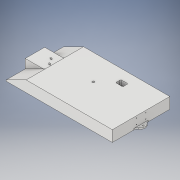
# Autodesk Inventor part: Enclosure_v2
Saved by Autodesk Inventor 2019 (Build 230136000, 136)
## iProperties
Created: 2020-02-14
Part Number: Enclosure_v2
Material: Generic
Document SubType Name: Modeling
Designer: close
Density: 1 g/cm^3
Appearance: Smooth - White
Author: close
Autodesk Inventor part; units mm, degrees
ref_plane "YZ Plane" through (0, 0, 0) normal (1, 0, 0) x (0, 1, 0)
ref_plane "XZ Plane" through (0, 0, 0) normal (0, 1, 0) x (-1, 0, 0)
ref_plane "XY Plane" through (0, 0, 0) normal (0, 0, 1) x (1, 0, 0)
sketch "Sketch1" plane through (0, 0, 0) normal (0, 1, 0) x (-1, 0, 0)
  line L0 (0, 0) -> (240, 0)
  line L1 (240, 0) -> (240, -130)
  line L2 (240, -130) -> (0, -130)
  line L3 (0, -130) -> (0, 0)
  dimension "d0" = 130
  dimension "d1" = 240
  constraints: 8 end point, 2 parallel, 1 horizontal, 1 perpendicular
  measures "d0" distance between parallel lines of L2 L0
  measures "d1" distance between parallel lines of L3 L1
extrude "Main Rectangular Prism" add sketch "Sketch1" along normal blind 25
sketch "Sketch2" plane through (0, 0, 0) normal (0, -1, 0) x (1, 0, 0)
  line L0 (-5, -111) -> (-105, -111) construction
  line L1 (-105, -111) -> (-105, -32) construction
  line L2 (-105, -32) -> (-5, -32) construction
  line L3 (-5, -32) -> (-5, -111) construction
  line L4 (-15, -94) -> (-101, -94) construction
  line L5 (-101, -94) -> (-101, -36) construction
  line L6 (-101, -36) -> (-15, -36) construction
  line L7 (-15, -36) -> (-15, -94) construction
  line L8 (-103.25, -76.2) -> (-99.35, -76.2) construction
  line L9 (-99.35, -76.2) -> (-99.35, -53.8) construction
  line L10 (-99.35, -53.8) -> (-103.25, -53.8) construction
  line L11 (-103.25, -53.8) -> (-103.25, -76.2) construction
  line L12 (0, 0) -> (-240, 0) construction
  line L13 (-240, -130) -> (0, -130) construction
  line L14 (-2.5, -113) -> (-107.5, -113)
  line L15 (-107.5, -113) -> (-107.5, -29)
  line L16 (-107.5, -29) -> (-2.5, -29)
  line L17 (-2.5, -29) -> (-2.5, -113)
  line L18 (0, -130) -> (0, 0) projected
  dimension "d5" = 100
  dimension "d6" = 86
  dimension "d7" = 58
  dimension "d8" = 79
  dimension "d9" = 4
  dimension "d10" = 4
  dimension "d12" = 22.4
  dimension "d13" = 17.8
  dimension "d14" = 130
  dimension "d16" = 53.8
  dimension "d17" = 3.9
  dimension "d18" = 1.75
  dimension "d19" = 105
  dimension "d20" = 2.5
  dimension "d21" = 84
  dimension "d22" = 2
  dimension "d25" = 2.5
  constraints: 32 end point, 8 parallel, 4 horizontal, 4 perpendicular
  measures "d5" distance of L0.start L0.end
  measures "d6" distance of L4.start L4.end
  measures "d7" distance of L6.end L4.start
  measures "d8" distance of L2.end L0.start
  measures "d9" distance between parallel lines of L2 L6
  measures "d10" distance between parallel lines of L1 L5
  measures "d12" distance between parallel lines of L10 L8
  measures "d13" distance from line of L5.end L10
  measures "d14" distance between parallel lines of L12 L13
  measures "d16" distance between parallel lines of L13 L8
  measures "d17" distance between parallel lines of L11 L9
  measures "d18" distance between parallel lines of L1 L11
  measures "d19" distance of L14.start L14.end
  measures "d20" distance between parallel lines of L18 L17
  measures "d21" distance between parallel lines of L16 L14
  measures "d22" distance between parallel lines of L0 L14
  measures "d25" distance between parallel lines of L17 L3
sketch "Sketch21" plane through (0, 0, 0) normal (0, -1, 0) x (1, 0, 0)
  line L0 (5, -65) -> (-228, -65) construction
  line L1 (-228, -81) -> (-228, -49) construction
  line L2 (-240, -130) -> (0, -130) construction
  line L3 (0, 0) -> (-240, 0) construction
  line L4 (-240, 0) -> (-240, -130) construction
  dimension "d221" = 233
  dimension "d222" = 32
  dimension "d223" = 130
  dimension "d224" = 65
  dimension "d225" = 12
  constraints: 4 end point, 1 horizontal, 1 midpoint, 1 vertical
  measures "d221" distance of L0.start L0.end
  measures "d222" distance of L1.end L1.start
  measures "d223" distance between parallel lines of L2 L3
  measures "d224" distance from line of L0.start L2
  measures "d225" distance between parallel lines of L4 L1
sketch "Sketch22" plane through (0, 25, 0) normal (0, 1, 0) x (1, 0, 0)
  line L0 (-240, 0) -> (-240, 130) projected
  line L1 (-195, 0) -> (-195, 130) projected
  line L2 (-240, 87) -> (-195, 87)
  line L3 (-195, 87) -> (-195, 43)
  line L4 (-195, 43) -> (-240, 43)
  line L5 (-240, 43) -> (-240, 87)
  line L6 (-195, 130) -> (-240, 130) projected
  point P0 (0, 0)
  dimension "d226" = 44
  dimension "d227" = 130
  dimension "d228" = 43
  constraints: 8 end point, 2 parallel, 2 point on line, 1 horizontal, 1 perpendicular
  measures "d226" distance between parallel lines of L4 L2
  measures "d227" distance of L0.start L0.end
  measures "d228" distance between parallel lines of L2 L6
extrude "2mm indent" cut sketch "Sketch22" against normal blind 2 contours L0 L2 L1 L4
sketch "Sketch23" plane through (0, 0, 0) normal (0, -1, 0) x (1, 0, 0)
  line L0 (0, 0) -> (0, -130) projected
  arc A0 (0, -76.619) -> (0, -53.381) centre (-3, -65) ccw
  line L1 (-240, -130) -> (0, -130) projected
  point P0 (0, -115)
  dimension "d231" = 65
  dimension "d232" = 3
  dimension "d233" = 12
  constraints: 2 point on circle, 2 point on line, 1 centre point
  measures "d231" distance from line of L1 A0.centre
  measures "d232" distance from line of L0 A0.centre
  measures "d233" radius of A0
extrude "Extrusion26" add sketch "Sketch23" against normal blind 3
fillet "Rear mount fillet" radius 7 2 edges at (0, 1.5, -76.619) (0, 1.5, -53.381)
sketch "Sketch45" plane through (-240, 0, 0) normal (0, 0, 1) x (1, 0, 0)
  line L0 (45, 25) -> (0, 2.5)
  line L1 (0, 0) -> (0, 25) projected
  line L2 (0, 25) -> (0, 2.5)
  line L3 (0, 25) -> (240, 25) projected
  line L4 (45, 25) -> (0, 25)
  point P0 (240, 0)
  dimension "d590" = 2.5
  constraints: 6 end point, 2 collinear, 1 point on line
  measures "d590" distance of L1.start L0.end
extrude "Slope Left" cut sketch "Sketch45" against normal up to surface (43 mm away)
sketch "Sketch46" plane through (0, 0, -130) normal (0, 0, -1) x (-1, 0, 0)
  line L0 (195, 25) -> (240, 25) projected
  line L1 (240, 0) -> (240, 25) projected
  line L2 (195, 25) -> (240, 2.5) projected
  point P0 (0, 0)
extrude "Slope Right" cut sketch "Sketch46" against normal up to surface (43 mm away)
hole "Hole5" at (5, 0, -65) at (-228, 0, -81) at (-228, 0, -49) direction (0, 1, 0) diameter 3.4 depth 8.8 clearance for "Flat Head Machine Screw" size "M3" standard "Ansi Metric M Profile"
sketch "Sketch24" plane through (0, 23, 0) normal (0, 1, 0) x (1, 0, 0)
  line L0 (-201.625, 59) -> (-199.375, 59) construction
  line L1 (-201.625, 60.125) -> (-199.375, 60.125)
  line L2 (-199.375, 57.875) -> (-201.625, 57.875)
  arc A0 (-201.625, 60.125) -> (-201.625, 57.875) centre (-201.625, 59) ccw
  arc A1 (-199.375, 57.875) -> (-199.375, 60.125) centre (-199.375, 59) ccw
  line L3 (-208.375, 71) -> (-210.625, 71) construction
  line L4 (-208.375, 72.125) -> (-210.625, 72.125)
  line L5 (-210.625, 69.875) -> (-208.375, 69.875)
  arc A2 (-208.375, 69.875) -> (-208.375, 72.125) centre (-208.375, 71) ccw
  arc A3 (-210.625, 72.125) -> (-210.625, 69.875) centre (-210.625, 71) ccw
  line L6 (-195, 87) -> (-195, 43) projected
  circle A4 centre (5, 65) radius 1.7 projected
  point P0 (0, 0)
  point P1 (-205, 65)
  point P2 (-200.5, 59)
  point P3 (-209.5, 71)
  dimension "d244" = 2.25
  dimension "d245" = 2.25
  dimension "d246" = 2.25
  dimension "d247" = 2.25
  dimension "d248" = 12
  dimension "d249" = 6
  dimension "d250" = 9
  dimension "d251" = 4.5
  dimension "d255" = 10
  dimension "d589" = 210
  constraints: 16 end point, 8 point on circle, 8 tangent, 4 centre point, 3 parallel, 2 midpoint, 1 horizontal
  measures "d244" distance of L3.start L3.end
  measures "d245" distance of L0.start L0.end
  measures "d246" distance between parallel lines of L2 L1
  measures "d247" distance between parallel lines of L5 L4
  measures "d248" distance between parallel lines of L0 L3
  measures "d249" distance from line of point (-205, 65) L0
  measures "d250" horizontal distance of point (-209.5, 71) point (-200.5, 59)
  measures "d251" horizontal distance of point (-200.5, 59) point (-205, 65)
  measures "d255" distance from line of L6 point (-205, 65)
  measures "d589" distance of A4.centre point (-205, 65)
extrude "Extrusion27" add sketch "Sketch24" along normal blind 2 contours L1 A1 L2 A0 | A2 L5 A3 L4
shell "Shell1" [suppressed]
sketch "Sketch27" plane through (-192.7649, 23, -128) normal (0, -1, 0) x (1, 0, 0)
  line L0 (186.2649, 18.5) -> (100.2649, 18.5) construction
  line L1 (100.2649, 18.5) -> (100.2649, 76.5) construction
  line L2 (100.2649, 76.5) -> (186.2649, 76.5) construction
  line L3 (186.2649, 76.5) -> (186.2649, 18.5) construction
  line L4 (190.2649, 1.5) -> (90.2649, 1.5) construction
  line L5 (90.2649, 1.5) -> (90.2649, 80.5) construction
  line L6 (90.2649, 80.5) -> (190.2649, 80.5) construction
  line L7 (190.2649, 80.5) -> (190.2649, 1.5) construction
  line L8 (60.9002, 126.8579) -> (96.9002, 126.8579) construction
  line L9 (38.0929, 36.45) -> (10.1929, 36.45) construction
  line L10 (190.7649, 0) -> (-45.2351, 0) construction
  line L11 (190.7649, 46.8445) -> (190.7649, 0) construction
  circle A0 centre (186.2649, 18.5) radius 3
  circle A1 centre (100.2649, 18.5) radius 3
  circle A2 centre (186.2649, 76.5) radius 3
  circle A3 centre (100.2649, 76.5) radius 3
  line L12 (186.2649, 15.5) -> (190.7649, 15.5)
  line L13 (186.2649, 21.5) -> (190.7649, 21.5)
  line L14 (190.7649, 15.5) -> (190.7649, 21.5)
  line L15 (186.2649, 73.5) -> (190.7649, 73.5)
  line L16 (190.7649, 126) -> (190.7649, 0) projected
  line L17 (186.2649, 79.5) -> (190.7649, 79.5)
  line L18 (190.7649, 73.5) -> (190.7649, 79.5)
  line L19 (192.7649, 79.1555) -> (192.7649, 128) projected
  point P0 (53.2929, 87.25)
  point P1 (5.0929, 88.55)
  point P2 (38.0929, 36.45)
  point P3 (-1.349, 0)
  point P4 (0.8663, 0)
  dimension "d288" = 100
  dimension "d289" = 79
  dimension "d290" = 86
  dimension "d291" = 58
  dimension "d298" = 1.3
  dimension "d299" = 27.9
  dimension "d300" = 5.1
  dimension "d301" = 50.8
  dimension "d303" = 4
  dimension "d304" = 4
  dimension "d305" = 1.5
  dimension "d306" = 0.5
  dimension "d307" = 6
  dimension "d309" = 6
  dimension "d310" = 6
  dimension "d556" = 187.672
  dimension "d557" = 6
  dimension "d564" = 15.2
  dimension "d565" = 88.55
  constraints: 32 end point, 10 coincident, 6 perpendicular, 6 point on line, 5 parallel, 4 centre point, 4 point on circle, 3 horizontal, 3 tangent, 1 collinear
  measures "d288" distance of L4.start L4.end
  measures "d289" distance of L6.end L4.start
  measures "d290" distance of L0.start L0.end
  measures "d291" distance of L2.end L0.start
  measures "d298" vertical distance of point (5.093, 88.55) point (53.293, 87.25)
  measures "d299" distance of L9.start L9.end
  measures "d300" horizontal distance of point (5.093, 88.55) point (10.193, 36.45)
  measures "d301" vertical distance of point (38.093, 36.45) point (53.293, 87.25)
  measures "d303" distance between parallel lines of L7 L3
  measures "d304" distance between parallel lines of L6 L2
  measures "d305" distance between parallel lines of L10 L4
  measures "d306" distance between parallel lines of L11 L7
  measures "d307" diameter of A0
  measures "d309" diameter of A2
  measures "d310" diameter of A3
  measures "d556" distance from line of L19 point (5.093, 88.55)
  measures "d557" diameter of A1
  measures "d564" horizontal distance of point (38.093, 36.45) point (53.293, 87.25)
  measures "d565" distance from line of L10 point (5.093, 88.55)
extrude "Extrusion30" [suppressed]
sketch "Sketch28" plane through (-192.7649, 3, -128) normal (0, -1, 0) x (1, 0, 0)
  arc A0 (186.2649, 21.5) -> (186.2649, 15.5) centre (186.2649, 18.5) ccw construction
  arc A1 (186.2649, 79.5) -> (186.2649, 73.5) centre (186.2649, 76.5) ccw construction
  circle A2 centre (100.2649, 76.5) radius 3 construction
  circle A3 centre (100.2649, 18.5) radius 3 construction
  arc A4 (186.2649, 79.5) -> (186.2649, 73.5) centre (186.2649, 76.5) ccw construction
  circle A5 centre (100.2649, 18.5) radius 3 construction
  point P0 (192.7649, 128)
  point P1 (186.2649, 18.5)
  point P2 (100.2649, 18.5)
  constraints: 4 coincident
hole "Hole7" [suppressed]
sketch "Sketch29" plane through (0, 25, 0) normal (0, 1, 0) x (1, 0, 0)
  line L0 (-81, 47.55) -> (-20, 47.55)
  line L1 (-20, 47.55) -> (-20, 88.55)
  line L2 (-81, 88.55) -> (-81, 47.55)
  line L3 (-79.85, 48.5) -> (-21.15, 48.5) construction
  line L4 (-21.15, 87.6) -> (-79.85, 87.6) construction
  line L5 (-79.85, 87.6) -> (-79.85, 80.3462) construction
  line L6 (-21.15, 87.6) -> (-21.15, 80.3462) construction
  line L7 (-5.3, 69.5) -> (-8.15, 69.5)
  line L8 (-8.15, 91.5) -> (-5.3, 91.5)
  line L9 (-8.15, 69.5) -> (-8.15, 91.5)
  line L10 (-5.3, 91.5) -> (-5.3, 69.5)
  line L11 (-66, 91.55) -> (-66, 91.55)
  line L12 (-63.8038, 91.55) -> (-58.1962, 91.55)
  line L13 (-56, 91.55) -> (-56, 91.55)
  line L14 (-20, 88.55) -> (-53, 88.55)
  line L15 (-69, 88.55) -> (-81, 88.55)
  arc A0 (-55.5981, 90.05) -> (-53, 88.55) centre (-53, 91.55) ccw
  arc A1 (-69, 88.55) -> (-66.4019, 90.05) centre (-69, 91.55) ccw
  arc A2 (-63.8038, 91.55) -> (-66.4019, 90.05) centre (-63.8038, 88.55) ccw
  arc A3 (-55.5981, 90.05) -> (-58.1962, 91.55) centre (-58.1962, 88.55) ccw
  point P0 (0, 0)
  dimension "d323" = 41
  dimension "d320" = 39.1
  dimension "d321" = 58.7
  dimension "d322" = 61
  dimension "d324" = 0.95
  dimension "d325" = 1.15
  dimension "d558" = 41
  dimension "d559" = 41
  dimension "d560" = 3
  dimension "d561" = 10
  dimension "d562" = 15
  dimension "d563" = 3
  constraints: 32 end point, 10 point on circle, 8 tangent, 5 horizontal, 5 parallel, 4 centre point, 3 equal radius, 3 vertical, 2 point on line, 1 perpendicular, 10 other
  measures "d320" distance between parallel lines of L4 L3
  measures "d321" distance of L4.start L4.end
  measures "d322" distance of L1.end L2.start
  measures "d324" distance between parallel lines of L3 L0
  measures "d325" distance between parallel lines of L5 L2
  measures "d558" distance between parallel lines of L0 L14
  measures "d559" distance between parallel lines of L0 L15
  measures "d560" distance between parallel lines of L15 L12
  measures "d561" distance of L11.end L13.start
  measures "d562" distance between parallel lines of L2 L11
  measures "d563" radius of A0
extrude "Extrusion31" [suppressed]
fillet "Fillet5" [suppressed]
sketch "Sketch30" plane through (0, 0, -130) normal (1, 0, 0) x (0, 0, -1)
  line L0 (-77.5, 31) -> (-52.5, 31) construction
  line L1 (-52.5, 31) -> (-52.5, 6) construction
  line L2 (-52.5, 6) -> (-77.5, 6) construction
  line L3 (-77.5, 6) -> (-77.5, 31) construction
  line L4 (-75.5, 20.5) -> (-54.5, 20.5) construction
  line L5 (-54.5, 20.5) -> (-54.5, 8) construction
  line L6 (-54.5, 8) -> (-75.5, 8) construction
  line L7 (-75.5, 8) -> (-75.5, 20.5) construction
  line L8 (-130, 25) -> (0, 25) construction
  line L9 (0, 0) -> (0, 25) construction
  line L10 (-130, 0) -> (-130, 25) construction
  line L11 (-72, 23) -> (-58, 23)
  line L12 (-56, 21) -> (-56, 11)
  line L13 (-58, 9) -> (-72, 9)
  line L14 (-74, 11) -> (-74, 21)
  arc A0 (-72, 23) -> (-74, 21) centre (-72, 21) ccw
  arc A1 (-74, 11) -> (-72, 9) centre (-72, 11) ccw
  arc A2 (-58, 9) -> (-56, 11) centre (-58, 11) ccw
  arc A3 (-56, 21) -> (-58, 23) centre (-58, 21) ccw
  point P0 (-74, 23)
  point P1 (-56, 9)
  point P2 (-56, 23)
  point P3 (-74, 9)
  dimension "d329" = 25
  dimension "d330" = 25
  dimension "d331" = 6
  dimension "d332" = 12.5
  dimension "d333" = 21
  dimension "d334" = 2
  dimension "d335" = 2
  dimension "d336" = 130
  dimension "d337" = 52.5
  dimension "d338" = 18
  dimension "d339" = 14
  dimension "d340" = 3.5
  dimension "d341" = 8
  dimension "d351" = 2
  constraints: 24 end point, 8 point on circle, 8 point on line, 8 tangent, 6 parallel, 4 centre point, 4 coincident, 3 equal radius, 3 horizontal, 3 perpendicular
  measures "d329" distance of L0.end L1.end
  measures "d330" distance of L0.start L0.end
  measures "d331" distance between parallel lines of L8 L0
  measures "d332" distance of L4.end L5.end
  measures "d333" distance of L5.end L6.end
  measures "d334" distance between parallel lines of L1 L5
  measures "d335" distance between parallel lines of L2 L6
  measures "d336" distance between parallel lines of L9 L10
  measures "d337" distance between parallel lines of L3 L10
  measures "d338" distance of point (-74, 23) point (-56, 23)
  measures "d339" distance between parallel lines of L13 L11
  measures "d340" distance between parallel lines of L3 L14
  measures "d341" distance between parallel lines of L0 L11
  measures "d351" radius of A0
extrude "Extrusion32" [suppressed]
hole "Hole8" at (0, 20.5, -54.5) at (0, 8, -54.5) at (0, 8, -75.5) at (0, 20.5, -75.5) direction (-1, 0, 0) diameter 1.567 depth 6.3 thread size "M2x0.4" class "6H" standard "ANSI Metric M Profile"
sketch "Sketch31" plane through (-194.1139, 0, -128) normal (0, 0, 1) x (1, 0, 0)
  line L0 (-43.8861, 23) -> (192.1139, 23) construction
  line L1 (192.1139, 0) -> (192.1139, 23) construction
  line L2 (-43.8861, 0) -> (192.1139, 0) construction
  circle A0 centre (185.5918, 9.5024) radius 3
  arc A1 (122.6139, 16.45) -> (122.4139, 16.65) centre (122.4139, 16.45) ccw construction
  line L3 (106.7139, 16.4) -> (106.7139, 3.35)
  line L4 (122.6139, 16.45) -> (122.6139, 16.6499)
  line L5 (122.6139, 16.6499) -> (122.4139, 16.65)
  line L6 (122.6139, 16.6499) -> (106.7139, 16.6499)
  line L7 (106.7139, 16.6499) -> (106.7139, 3.35)
  line L8 (106.7139, 3.35) -> (122.6139, 3.35)
  line L9 (122.6139, 3.35) -> (122.6139, 16.6499)
  arc A2 (126.0639, 18.47) -> (125.4639, 17.87) centre (126.0639, 17.87) ccw construction
  arc A3 (125.4639, 4.85) -> (126.0639, 4.25) centre (126.0639, 4.85) ccw construction
  arc A4 (138.5639, 17.87) -> (137.9639, 18.47) centre (137.9639, 17.87) ccw construction
  line L10 (138.5639, 17.87) -> (138.5639, 18.47) construction
  line L11 (138.5639, 18.47) -> (137.9639, 18.47) construction
  line L12 (126.0639, 18.47) -> (125.4639, 18.47) construction
  line L13 (125.4639, 18.47) -> (125.4639, 17.87) construction
  line L14 (125.4639, 4.85) -> (125.4639, 4.25) construction
  line L15 (125.4639, 4.25) -> (126.0639, 4.25) construction
  line L16 (138.5639, 18.47) -> (125.4639, 18.47)
  line L17 (125.4639, 18.47) -> (125.4639, 12.75)
  line L18 (125.4639, 12.75) -> (138.5639, 12.75)
  line L19 (138.5639, 12.75) -> (138.5639, 18.47)
  line L20 (155.5639, 12.75) -> (155.5639, 18.47)
  line L21 (155.5639, 18.47) -> (142.4639, 18.47)
  line L22 (142.4639, 18.47) -> (142.4639, 12.75)
  line L23 (142.4639, 12.75) -> (155.5639, 12.75)
  line L24 (138.5639, 4.25) -> (138.5639, 9.97)
  line L25 (138.5639, 9.97) -> (125.4639, 9.97)
  line L26 (125.4639, 9.97) -> (125.4639, 4.25)
  line L27 (125.4639, 4.25) -> (138.5639, 4.25)
  line L28 (155.5639, 4.25) -> (155.5639, 9.97)
  line L29 (155.5639, 9.97) -> (142.4639, 9.97)
  line L30 (142.4639, 9.97) -> (142.4639, 4.25)
  line L31 (142.4639, 4.25) -> (155.5639, 4.25)
  arc A5 (176.3139, 20.3762) -> (175.5139, 21.1762) centre (175.5139, 20.3762) ccw
  arc A6 (176.1088, 17.2149) -> (176.31, 17.6362) centre (175.6139, 17.7099) ccw
  arc A7 (160.2139, 21.1762) -> (159.4201, 20.4762) centre (160.2139, 20.3762) ccw
  line L32 (175.5139, 21.1762) -> (160.2139, 21.1762)
  arc A8 (159.4211, 16.2162) -> (160.1139, 15.6162) centre (160.1139, 16.3162) ccw
  arc A9 (174.2102, 15.6062) -> (174.7051, 15.8112) centre (174.2102, 16.3062) ccw
  line L33 (176.31, 17.6362) -> (176.3139, 20.3762)
  line L34 (176.1088, 17.2149) -> (174.7051, 15.8112)
  line L35 (174.2102, 15.6062) -> (160.1139, 15.6162)
  line L36 (159.4211, 16.2162) -> (159.4201, 20.4762)
  line L37 (-43.8861, 23) -> (192.1139, 23) projected
  line L38 (192.1139, 0) -> (192.1139, 23) projected
  line L39 (-43.8861, 0) -> (192.1139, 0) projected
  arc A10 (175.3629, 8.3762) -> (174.5629, 9.1762) centre (174.5629, 8.3762) ccw
  arc A11 (161.1629, 9.1762) -> (160.3629, 8.3762) centre (161.1629, 8.3762) ccw
  arc A12 (160.3629, 5.8978) -> (160.9276, 5.1331) centre (161.1629, 5.8978) ccw
  arc A13 (161.6118, 4.8762) -> (161.4748, 4.9648) centre (161.3866, 4.678) ccw
  arc A14 (162.4729, 3.8977) -> (163.0735, 3.6262) centre (163.0735, 4.4262) ccw
  arc A15 (172.6523, 3.6262) -> (173.2528, 3.8977) centre (172.6523, 4.4262) ccw
  arc A16 (174.2509, 4.9648) -> (174.1139, 4.8762) centre (174.3391, 4.678) ccw
  arc A17 (174.7981, 5.1331) -> (175.3629, 5.8978) centre (174.5629, 5.8978) ccw
  line L40 (174.5629, 9.1762) -> (161.1629, 9.1762)
  line L41 (160.3629, 8.3762) -> (160.3629, 5.8978)
  line L42 (160.9276, 5.1331) -> (161.4748, 4.9648)
  line L43 (161.6118, 4.8762) -> (162.4729, 3.8977)
  line L44 (163.0735, 3.6262) -> (172.6523, 3.6262)
  line L45 (174.1139, 4.8762) -> (173.2528, 3.8977)
  line L46 (174.7981, 5.1331) -> (174.2509, 4.9648)
  line L47 (175.3629, 8.3762) -> (175.3629, 5.8978)
  line L48 (-43.8861, 0) -> (-43.8861, 23) projected
  line L49 (-43.8861, 0) -> (-43.8861, 23) projected
  point P0 (194.1139, 0)
  dimension "d360" = 6
  dimension "d416" = 6.5221
  dimension "d473" = 17
  dimension "d476" = 8.5
  dimension "d479" = 0
  constraints: 84 end point, 34 point on circle, 18 centre point, 9 perpendicular, 9 tangent, 6 horizontal, 4 parallel, 3 vertical, 2 collinear, 1 point on line, 92 other
  measures "d360" diameter of A0
  measures "d416" distance from line of A0.centre L1
  measures "d473" distance of L18.end L20.start
  measures "d476" distance of L18.end L24.start
  measures "d479" distance between parallel lines of L15 L27
extrude "Extrusion33" [suppressed]
sketch "Sketch32" plane through (0, 25, 0) normal (0, 1, 0) x (1, 0, 0)
  line L0 (-74.17, 95.83) -> (-86.33, 95.83)
  line L1 (-88.33, 97.83) -> (-88.33, 105.63)
  line L2 (-86.33, 107.63) -> (-74.17, 107.63)
  line L3 (-72.17, 105.63) -> (-72.17, 97.83)
  arc A0 (-74.17, 95.83) -> (-72.17, 97.83) centre (-74.17, 97.83) ccw
  arc A1 (-72.17, 105.63) -> (-74.17, 107.63) centre (-74.17, 105.63) ccw
  arc A2 (-86.33, 107.63) -> (-88.33, 105.63) centre (-86.33, 105.63) ccw
  arc A3 (-88.33, 97.83) -> (-86.33, 95.83) centre (-86.33, 97.83) ccw
  point P0 (0, 0)
  point P1 (-75.17, 104.63)
  point P2 (-85.33, 104.63)
  point P3 (-85.33, 98.83)
  point P4 (-75.17, 98.83)
  dimension "d480" = 2
  dimension "d481" = 3
  dimension "d482" = 3
  dimension "d483" = 3
  dimension "d484" = 3
  constraints: 8 end point, 8 point on circle, 8 tangent, 4 centre point, 3 equal radius, 2 parallel, 1 horizontal, 1 perpendicular, 4 other
  measures "d480" radius of A0
  measures "d481" distance from line of L3 point (-75.17, 98.83)
  measures "d482" distance from line of point (-85.33, 98.83) L0
  measures "d483" distance from line of point (-85.33, 98.83) L1
  measures "d484" distance from line of L2 point (-85.33, 104.63)
extrude "Extrusion34" cut sketch "Sketch32" against normal blind 10
sketch "Sketch33" plane through (0, 25, 0) normal (0, 1, 0) x (1, 0, 0)
  circle A0 centre (-128.5, 111.25) radius 1.2295 construction
  circle A1 centre (-99.5, 111.25) radius 1.2295 construction
  circle A2 centre (-99.5, 58.75) radius 1.2295 construction
  circle A3 centre (-128.5, 58.75) radius 1.2295 construction
  circle A4 centre (-102.1923, 37.5) radius 2.25 construction
  circle A5 centre (-102.1923, 6) radius 2.25 construction
  circle A6 centre (-7.1923, 37.5) radius 2.25 construction
  circle A7 centre (-7.1923, 6) radius 2.25 construction
  circle A8 centre (-126.2337, 102.7663) radius 1.7399 construction
  circle A9 centre (-126.2337, 67.4838) radius 1.7399 construction
  circle A10 centre (-115.03, 72.27) radius 1.095 construction
  line L0 (-117.7, 74) -> (-131.7, 74)
  line L1 (-131.7, 74) -> (-131.7, 96.5)
  line L2 (-131.7, 96.5) -> (-117.7, 96.5)
  line L3 (-117.7, 96.5) -> (-117.7, 74)
  circle A11 centre (-126.2337, 67.4838) radius 2.5
  circle A12 centre (-115.03, 72.27) radius 2.5
  circle A13 centre (-22.5336, 9.0163) radius 1.7399 construction
  circle A14 centre (-39.5661, 9.0163) radius 1.7399 construction
  circle A15 centre (-56.5986, 9.0163) radius 1.7399 construction
  circle A16 centre (-73.6311, 9.0163) radius 1.7399 construction
  circle A17 centre (-73.6311, 9.0163) radius 2.5
  circle A18 centre (-56.5986, 9.0163) radius 2.5
  circle A19 centre (-39.5661, 9.0163) radius 2.5
  circle A20 centre (-22.5336, 9.0163) radius 2.5
  circle A21 centre (-126.2337, 102.7663) radius 2.5
  arc A22 (-76.7056, 21.95) -> (-76.4056, 21.65) centre (-76.4056, 21.95) ccw construction
  arc A23 (-70.3173, 35.2) -> (-70.6173, 35.5) centre (-70.6173, 35.2) ccw construction
  line L4 (-77.2056, 35.2) -> (-77.2056, 21.95) construction
  line L5 (-60.2056, 35.2) -> (-60.2056, 21.95) construction
  line L6 (-70.6173, 35.5) -> (-70.3173, 35.5) construction
  line L7 (-70.3173, 35.5) -> (-70.3173, 35.2) construction
  line L8 (-76.7056, 21.95) -> (-76.7056, 21.65) construction
  line L9 (-76.7056, 21.65) -> (-76.4056, 21.65) construction
  line L10 (-70.3173, 35.5) -> (-76.7056, 35.5)
  line L11 (-76.7056, 35.5) -> (-76.7056, 21.65)
  line L12 (-76.7056, 21.65) -> (-70.3173, 21.65)
  line L13 (-70.3173, 21.65) -> (-70.3173, 35.5)
  line L14 (-59.7056, 21.65) -> (-53.3173, 21.65)
  line L15 (-59.7056, 21.65) -> (-59.4056, 21.65) construction
  line L16 (-59.7056, 21.95) -> (-59.7056, 21.65) construction
  arc A24 (-59.7056, 21.95) -> (-59.4056, 21.65) centre (-59.4056, 21.95) ccw construction
  line L17 (-59.7056, 35.5) -> (-59.7056, 21.65)
  line L18 (-53.3173, 21.65) -> (-53.3173, 35.5)
  line L19 (-53.6173, 35.5) -> (-53.3173, 35.5) construction
  line L20 (-53.3173, 35.5) -> (-53.3173, 35.2) construction
  arc A25 (-53.3173, 35.2) -> (-53.6173, 35.5) centre (-53.6173, 35.2) ccw construction
  line L21 (-53.3173, 35.5) -> (-59.7056, 35.5)
  line L22 (-42.7056, 21.65) -> (-36.3173, 21.65)
  line L23 (-42.7056, 21.65) -> (-42.4056, 21.65) construction
  line L24 (-42.7056, 21.95) -> (-42.7056, 21.65) construction
  arc A26 (-42.7056, 21.95) -> (-42.4056, 21.65) centre (-42.4056, 21.95) ccw construction
  line L25 (-42.7056, 35.5) -> (-42.7056, 21.65)
  line L26 (-36.3173, 21.65) -> (-36.3173, 35.5)
  line L27 (-36.6173, 35.5) -> (-36.3173, 35.5) construction
  line L28 (-36.3173, 35.5) -> (-36.3173, 35.2) construction
  arc A27 (-36.3173, 35.2) -> (-36.6173, 35.5) centre (-36.6173, 35.2) ccw construction
  line L29 (-36.3173, 35.5) -> (-42.7056, 35.5)
  line L30 (-25.7056, 21.65) -> (-19.3173, 21.65)
  line L31 (-25.7056, 21.65) -> (-25.4056, 21.65) construction
  line L32 (-25.7056, 21.95) -> (-25.7056, 21.65) construction
  arc A28 (-25.7056, 21.95) -> (-25.4056, 21.65) centre (-25.4056, 21.95) ccw construction
  line L33 (-25.7056, 35.5) -> (-25.7056, 21.65)
  line L34 (-19.3173, 21.65) -> (-19.3173, 35.5)
  line L35 (-19.6173, 35.5) -> (-19.3173, 35.5) construction
  line L36 (-19.3173, 35.5) -> (-19.3173, 35.2) construction
  arc A29 (-19.3173, 35.2) -> (-19.6173, 35.5) centre (-19.6173, 35.2) ccw construction
  line L37 (-19.3173, 35.5) -> (-25.7056, 35.5)
  point P0 (0, 0)
  dimension "d495" = 5
  dimension "d496" = 5
  dimension "d551" = 5
  dimension "d552" = 5
  dimension "d553" = 5
  dimension "d554" = 5
  dimension "d555" = 5
  dimension "d566" = 17
  dimension "d569" = 17
  constraints: 76 end point, 30 centre point, 16 point on circle, 7 coincident, 5 parallel, 4 horizontal, 4 perpendicular, 2 tangent, 2 vertical, 1 collinear, 103 other
  measures "d495" diameter of A11
  measures "d496" diameter of A12
  measures "d551" diameter of A17
  measures "d552" diameter of A18
  measures "d553" diameter of A19
  measures "d554" diameter of A20
  measures "d555" diameter of A21
  measures "d566" distance between parallel lines of L5 L4
  measures "d569" distance of L8.end L14.start
extrude "Extrusion35" [suppressed]
sketch "Sketch34" plane through (-192.4508, 23, -128) normal (0, -1, 0) x (1, 0, 0)
  line L0 (75.7508, 28.5) -> (57.7508, 28.5)
  line L1 (57.7508, 28.5) -> (57.7508, 57)
  line L2 (57.7508, 57) -> (75.7508, 57)
  line L3 (75.7508, 57) -> (75.7508, 28.5)
  line L4 (74.7508, 31.5) -> (60.7508, 31.5) projected
  line L5 (74.7508, 54) -> (74.7508, 31.5) projected
  line L6 (60.7508, 31.5) -> (60.7508, 54) projected
  line L7 (60.7508, 54) -> (74.7508, 54) projected
  point P0 (192.4508, 128)
  dimension "d499" = 3
  dimension "d500" = 1
  dimension "d501" = 3
  dimension "d502" = 3
  constraints: 8 end point, 2 parallel, 1 horizontal, 1 perpendicular
  measures "d499" distance between parallel lines of L0 L4
  measures "d500" distance between parallel lines of L5 L3
  measures "d501" distance between parallel lines of L1 L6
  measures "d502" distance between parallel lines of L2 L7
extrude "Extrusion36" [suppressed]
fillet "Fillet6" [suppressed]
extrude "Extrusion37" cut sketch "Sketch33" against normal through all contours A12
sketch "Sketch36" plane through (-192.4508, 23, -128) normal (0, -1, 0) x (1, 0, 0)
  circle A0 centre (185.2585, 90.5) radius 3
  circle A1 centre (90.2585, 90.5) radius 3
  circle A2 centre (185.2585, 122) radius 3
  circle A3 centre (90.2585, 122) radius 3
  circle A4 centre (52.9788, 87.25) radius 3
  circle A5 centre (4.7788, 88.55) radius 3
  circle A6 centre (9.8788, 36.45) radius 3
  circle A7 centre (37.7788, 36.45) radius 3
  circle A8 centre (63.9508, 69.25) radius 3
  circle A9 centre (92.9508, 69.25) radius 3
  circle A10 centre (92.9508, 16.75) radius 3
  circle A11 centre (63.9508, 16.75) radius 3
  point P0 (192.4508, 128)
  point P1 (63.9508, 16.75)
  point P2 (92.9508, 16.75)
  point P3 (90.2585, 122)
  point P4 (185.2585, 122)
  dimension "d508" = 6
  dimension "d509" = 6
  dimension "d510" = 6
  dimension "d511" = 6
  dimension "d512" = 6
  dimension "d513" = 6
  dimension "d514" = 6
  dimension "d515" = 6
  dimension "d516" = 6
  dimension "d517" = 6
  dimension "d518" = 6
  dimension "d519" = 6
  constraints: 12 centre point, 12 coincident
  measures "d508" diameter of A10
  measures "d509" diameter of A11
  measures "d510" diameter of A9
  measures "d511" diameter of A8
  measures "d512" diameter of A7
  measures "d513" diameter of A6
  measures "d514" diameter of A4
  measures "d515" diameter of A5
  measures "d516" diameter of A0
  measures "d517" diameter of A1
  measures "d518" diameter of A2
  measures "d519" diameter of A3
extrude "Extrusion38" [suppressed]
extrude "Extrusion39" [suppressed]
extrude "Extrusion40" [suppressed]
sketch "Sketch38" plane through (-102.1923, 8.5, -6) normal (0, -1, 0) x (1, 0, 0)
  circle A0 centre (0, 0) radius 3 construction
  circle A1 centre (0, -31.5) radius 3 construction
  circle A2 centre (95, -31.5) radius 3 construction
  circle A3 centre (95, 0) radius 3 construction
  point P0 (102.1923, 6)
  constraints: 4 coincident
hole "Hole9" [suppressed]
sketch "Sketch39" plane through (-128.5, 11, -58.75) normal (0, -1, 0) x (1, 0, 0)
  circle A0 centre (0, 0) radius 3 construction
  circle A1 centre (29, 0) radius 3 construction
  circle A2 centre (0, -52.5) radius 3 construction
  circle A3 centre (29, -52.5) radius 3 construction
  point P0 (128.5, 58.75)
  point P1 (29, -52.5)
  constraints: 4 coincident
hole "Hole10" [suppressed]
sketch "Sketch40" plane through (-187.672, 18.5, -39.45) normal (0, -1, 0) x (1, 0, 0)
  circle A0 centre (0, 0) radius 3 construction
  circle A1 centre (48.2, -1.3) radius 3 construction
  circle A2 centre (33, -52.1) radius 3 construction
  circle A3 centre (5.1, -52.1) radius 3 construction
  point P0 (187.672, 39.45)
  point P1 (48.2, -1.3)
  constraints: 4 coincident
hole "Hole11" [suppressed]
sketch "Sketch41" plane through (0, 0, -130) normal (1, 0, 0) x (0, 0, -1)
  arc A0 (-115.65, 9.3) -> (-115.35, 9) centre (-115.35, 9.3) ccw construction
  arc A1 (-101.8, 15.0999) -> (-102.1, 15.3999) centre (-102.1, 15.0999) ccw construction
  line L0 (-115.65, 9.3) -> (-115.65, 9) construction
  line L1 (-115.65, 9) -> (-115.35, 9) construction
  line L2 (-102.1, 15.3999) -> (-101.8, 15.3999) construction
  line L3 (-101.8, 15.3999) -> (-101.8, 15.0999) construction
  line L4 (-115.65, 9) -> (-101.8, 9)
  line L5 (-101.8, 9) -> (-101.8, 15.3999)
  line L6 (-101.8, 15.3999) -> (-115.65, 15.3999)
  line L7 (-115.65, 15.3999) -> (-115.65, 9)
  point P0 (-130, 0)
  constraints: 16 end point, 5 point on circle, 3 perpendicular, 2 centre point, 2 horizontal, 2 parallel, 1 tangent, 1 vertical, 8 other
extrude "Extrusion41" [suppressed]
fillet "Fillet8" [suppressed]
sketch "Sketch42" plane through (-192.4508, 23, -128) normal (0, -1, 0) x (1, 0, 0)
  line L0 (4.7989, 6) -> (4.7989, 120) construction
  line L1 (190.4508, 0) -> (-45.5492, 0) projected
  ellipse E0 centre (-1.2011, 6.9332) end of major axis (-5.932, 19.1912) minor radius 1.7347 (-3.0581, 6.9332) -> (-1.2011, 2.3748) ccw projected
  line L2 (-45.5492, 126) -> (190.4508, 126) projected
  point P0 (192.4508, 128)
  point P1 (-1.6631, 0)
  point P2 (0.5523, 126)
  point P3 (0.5523, 0)
  point P4 (-1.6631, 126)
  dimension "d582" = 6
  dimension "d583" = 6
  dimension "d584" = 6
  constraints: 2 coincident, 2 end point, 1 vertical, 1 other
  measures "d582" distance from line of L1 L0.start
  measures "d583" horizontal distance of point (-1.201, 6.933) L0.start
  measures "d584" distance from line of L2 point (4.799, 120)
hole "Hole12" [suppressed]
equation "\"d10\" = d9"
equation "\"d16\" = -0.5 * d12 + 0.5 * d14"
equation "\"d25\" = -0.5 * d5 + 0.5 * d19"
body "Solid1"
